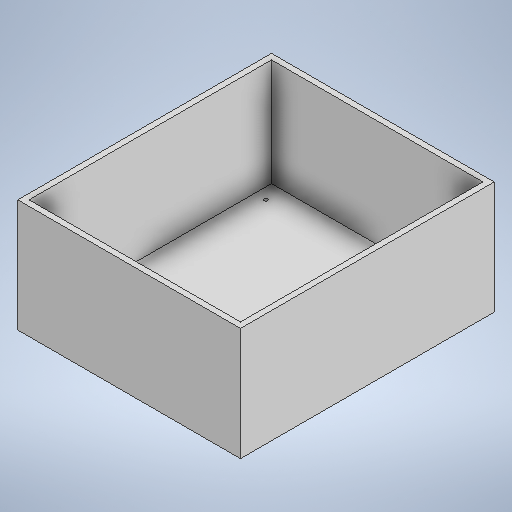
# Autodesk Inventor part: Box
Saved by Autodesk Inventor 2025.3 (Build 293356000, 356)
## iProperties
Created: 2026-04-19
Part Number: Box
Material: Generic
Document SubType Name: Modeling
Designer: ksawe
Density: 1 g/cm^3
Appearance: Default
Author: ksawe
Autodesk Inventor part; units mm, degrees
ref_plane "YZ Plane" through (0, 0, 0) normal (1, 0, 0) x (0, 1, 0)
ref_plane "XZ Plane" through (0, 0, 0) normal (0, 1, 0) x (-1, 0, 0)
ref_plane "XY Plane" through (0, 0, 0) normal (0, 0, 1) x (1, 0, 0)
sketch "Sketch1" plane through (0, 0, 0) normal (0, 1, 0) x (-1, 0, 0)
  line L0 (98.75, 112.5) -> (-98.75, 112.5)
  line L1 (-98.75, 112.5) -> (-98.75, -112.5)
  line L2 (-98.75, -112.5) -> (98.75, -112.5)
  line L3 (98.75, -112.5) -> (98.75, 112.5)
  line L4 (98.75, 112.5) -> (-98.75, -112.5) construction
  line L5 (-98.75, 112.5) -> (98.75, -112.5) construction
  point P0 (0, 0)
  dimension "d0" = 197.5
  dimension "d1" = 225
  constraints: 12 end point, 2 midpoint, 2 parallel, 1 horizontal, 1 perpendicular
  measures "d0" distance of L2.end L1.end
  measures "d1" distance of L1.end L0.end
extrude "Extrusion1" add sketch "Sketch1" along normal blind 100
shell "Shell1" thickness 5 removed faces 1 at (32.9167, 100, 37.5)
sketch "Sketch2" plane through (-93.75, 5, -107.5) normal (0, 1, 0) x (1, 0, 0)
  circle A0 centre (10, -15) radius 1.5
  line L0 (187.5, -215) -> (0, -215) projected
  line L1 (93.75, -215) -> (93.75, 0)
  line L2 (0, 0) -> (187.5, 0) projected
  line L3 (187.5, -215) -> (187.5, 0) projected
  line L4 (0, -215) -> (0, 0) projected
  line L5 (192.5, 5) -> (-5, 5) projected
  circle A1 centre (10, -205.267) radius 1.5
  circle A2 centre (177.5, -15) radius 1.5
  circle A3 centre (177.5, -205.267) radius 1.5
  point P0 (93.75, -107.5)
  dimension "d5" = 3
  dimension "d6" = 20
  dimension "d7" = 3
  dimension "d8" = 190.267
  dimension "d9" = 10
  constraints: 4 centre point, 2 end point, 2 midpoint, 2 symmetric about line, 1 vertical alignment, 2 other
  measures "d5" diameter of A0
  measures "d6" distance from line of L5 A0.centre
  measures "d7" diameter of A1
  measures "d8" distance of A0.centre A1.centre
  measures "d9" distance from line of L4 A0.centre
extrude "Extrusion2" cut sketch "Sketch2" against normal through all contours A0 | A1 | A2 | A3
body "Solid1"
